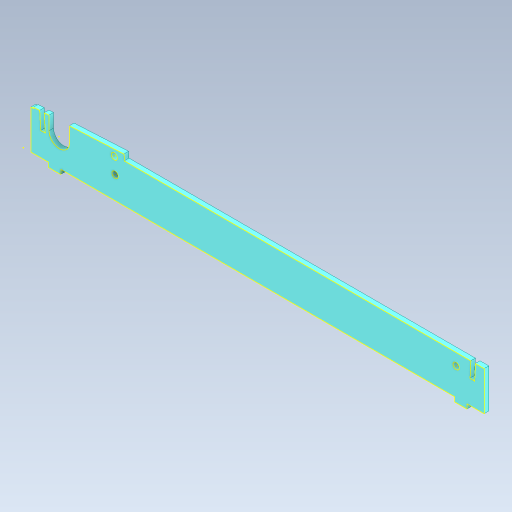
# Autodesk Inventor part: 零件1
Saved by Autodesk Inventor 2023 (Build 270158000, 158)
## iProperties
Created: 2023-04-16
Part Number: 零件1
Material: 一般
Document SubType Name: Modeling
Designer: JOU
Density: 1 g/cm^3
Appearance: 預設
Author: JOU
Autodesk Inventor part; units mm, degrees
ref_plane "YZ Plane" through (0, 0, 0) normal (1, 0, 0) x (0, 1, 0)
ref_plane "XZ Plane" through (0, 0, 0) normal (0, 1, 0) x (-1, 0, 0)
ref_plane "XY Plane" through (0, 0, 0) normal (0, 0, 1) x (1, 0, 0)
sketch "草圖1" plane through (0, 0, 0) normal (0, 0, 1) x (1, 0, 0)
  line L0 (0, 25) -> (300, 25)
  line L1 (300, 25) -> (300, 0)
  line L2 (300, 0) -> (0, 0)
  line L3 (0, 0) -> (0, 25)
  circle A0 centre (23, 17.5) radius 6.55
  circle A1 centre (277, 17.5) radius 2
  line L4 (16, 0) -> (24, 0)
  line L5 (24, 0) -> (24, -2.9)
  line L6 (24, -2.9) -> (16, -2.9)
  line L7 (16, -2.9) -> (16, 0)
  line L8 (276, 0) -> (284, 0)
  line L9 (284, 0) -> (284, -2.9)
  line L10 (284, -2.9) -> (276, -2.9)
  line L11 (276, -2.9) -> (276, 0)
  line L12 (0, 25) -> (5, 25)
  line L13 (5, 25) -> (5, 0)
  line L14 (5, 0) -> (0, 0)
  line L15 (0, 0) -> (0, 25)
  line L16 (300, 25) -> (295, 25)
  line L17 (295, 25) -> (295, 0)
  line L18 (295, 0) -> (300, 0)
  line L19 (300, 0) -> (300, 25)
  line L20 (24, -1.45) -> (276, -1.45) construction
  point P0 (16, -1.45)
  point P1 (284, -1.45)
  point P2 (284, 0)
  point P3 (24, 0)
  point P4 (150, -1.45)
  point P5 (150, 0)
  dimension "d0" = 300
  dimension "d1" = 25
  dimension "d2" = 7.5
  dimension "d3" = 13.1
  dimension "d4" = 23
  dimension "d5" = 23
  dimension "d6" = 7.5
  dimension "d7" = 4
  dimension "d12" = 8
  dimension "d13" = 2.9
  dimension "d14" = 8
  dimension "d30" = 5
  dimension "d31" = 5
  dimension "d32" = 252
  constraints: 42 end point, 10 parallel, 6 midpoint, 5 horizontal, 5 perpendicular, 5 point on line, 2 centre point, 1 coincident, 1 vertical alignment
  measures "d0" distance of L0.start L0.end
  measures "d1" distance of L2.end L0.start
  measures "d2" distance from line of L0 A0.centre
  measures "d3" diameter of A0
  measures "d4" distance from line of L3 A0.centre
  measures "d5" distance from line of A1.centre L1
  measures "d6" distance from line of L0 A1.centre
  measures "d7" diameter of A1
  measures "d12" distance of L5.end L6.end
  measures "d13" distance of L4.end L5.end
  measures "d14" distance of L9.end L10.end
  measures "d30" distance between parallel lines of L3 L13
  measures "d31" distance between parallel lines of L1 L17
  measures "d32" distance from line of L20.start L11
extrude "擠出1" add sketch "草圖1" along normal blind 3 contours L0 L17 L2 L13 | L2 L5 L6 L7 | L9 L10 L11 L2
sketch "草圖2" plane through (0, 0, 3) normal (0, 0, 1) x (1, 0, 0)
  line L0 (10.5404, 25) -> (13.4864, 25.1544)
  line L1 (13.4864, 25.1544) -> (14.0097, 15.1681)
  line L2 (14.0097, 15.1681) -> (11.0638, 15.0137)
  line L3 (11.0638, 15.0137) -> (10.5404, 25)
  line L4 (295, 25) -> (5, 25) projected
  line L5 (16.048, 25) -> (29.13, 25.6856)
  line L6 (29.13, 25.6856) -> (30.1465, 6.2887)
  line L7 (30.1465, 6.2887) -> (17.0645, 5.6031)
  line L8 (17.0645, 5.6031) -> (16.048, 25)
  circle A0 centre (23, 17.5) radius 6.55 projected
  line L9 (14.0097, 15.1681) -> (16.5562, 15.3016)
  line L10 (286.4135, 25.1544) -> (289.3595, 25)
  line L11 (289.3595, 25) -> (288.8361, 15.0137)
  line L12 (288.8361, 15.0137) -> (285.8901, 15.1681)
  line L13 (285.8901, 15.1681) -> (286.4135, 25.1544)
  line L14 (275.2453, 22.2337) -> (279.2399, 22.0243)
  line L15 (279.2399, 22.0243) -> (278.6818, 11.3762)
  line L16 (278.6818, 11.3762) -> (274.6873, 11.5855)
  line L17 (274.6873, 11.5855) -> (275.2453, 22.2337)
  circle A1 centre (277, 17.5) radius 2 projected
  line L18 (285.8901, 15.1681) -> (278.8997, 15.5344)
  point P0 (0, 0)
  point P1 (300, 25)
  point P2 (0, 25)
  point P3 (286.4054, 25)
  point P4 (13.4945, 25)
  dimension "d16" = 2.95
  dimension "d18" = 10
  dimension "d19" = 87
  dimension "d20" = 87
  dimension "d22" = 87
  dimension "d23" = 87
  dimension "d24" = 2.95
  dimension "d25" = 10
  dimension "d33" = 9.1
  dimension "d34" = 9
  constraints: 36 end point, 8 parallel, 6 perpendicular, 4 point on line, 4 tangent, 1 midpoint
  measures "d16" distance of L0.start L0.end
  measures "d18" distance of L0.end L1.end
  measures "d19" angle of L1 L4
  measures "d20" angle of L6 L4
  measures "d22" angle of L4 L17
  measures "d23" angle of L4 L13
  measures "d24" distance of L10.start L10.end
  measures "d25" distance of L10.end L11.end
  measures "d33" distance from line of L1 A0.centre
  measures "d34" distance from line of L13 A1.centre
extrude "擠出2" cut sketch "草圖2" against normal up to surface (3 mm away) contours L4 L1 L2 L3 | L11 L12 L13 L4
sketch "草圖7" plane through (0, 0, 3) normal (0, 0, 1) x (1, 0, 0)
  line L0 (64.4714, 28.6858) -> (65.4135, 10.7104)
  line L1 (65.4135, 10.7104) -> (7.493, 7.675)
  line L2 (7.493, 7.675) -> (6.5509, 25.6503)
  line L3 (6.5509, 25.6503) -> (64.4714, 28.6858)
  line L4 (13.4945, 25) -> (14.0097, 15.1681) projected
  circle A0 centre (23, 17.5) radius 6.55 projected
  line L5 (285.8901, 15.1681) -> (286.4054, 25) projected
  line L6 (286.4054, 25) -> (13.4945, 25) projected
  line L7 (13.4945, 25) -> (14.0097, 15.1681) projected
  line L8 (14.0097, 15.1681) -> (11.0638, 15.0137) projected
  line L9 (11.0638, 15.0137) -> (10.5404, 25) projected
  line L10 (10.5404, 25) -> (5, 25) projected
  line L11 (5, 25) -> (5, 0) projected
  line L12 (5, 0) -> (16, 0) projected
  line L13 (16, 0) -> (16, -2.9) projected
  line L14 (16, -2.9) -> (24, -2.9) projected
  line L15 (24, -2.9) -> (24, 0) projected
  line L16 (24, 0) -> (276, 0) projected
  line L17 (276, 0) -> (276, -2.9) projected
  line L18 (276, -2.9) -> (284, -2.9) projected
  line L19 (284, -2.9) -> (284, 0) projected
  line L20 (284, 0) -> (295, 0) projected
  line L21 (295, 0) -> (295, 25) projected
  line L22 (295, 25) -> (289.3595, 25) projected
  line L23 (289.3595, 25) -> (288.8361, 15.0137) projected
  line L24 (288.8361, 15.0137) -> (285.8901, 15.1681) projected
  circle A1 centre (23, 17.5) radius 6.55 projected
  circle A2 centre (277, 17.5) radius 2 projected
  line L25 (13.4945, 25) -> (13.4414, 26.0114)
  line L26 (10.5404, 25) -> (11.0638, 15.0137) projected
  line L27 (10.5404, 25) -> (10.4955, 25.857)
  point P0 (0, 0)
  point P1 (64.6646, 25)
  point P2 (6.585, 25)
  dimension "d50" = 42
  dimension "d51" = 16
  dimension "d52" = 18
  dimension "d53" = 9
  constraints: 12 end point, 4 parallel, 2 point on line, 1 collinear, 1 perpendicular
  measures "d50" distance from line of L0 A0.centre
  measures "d51" distance from line of L2 A0.centre
  measures "d52" distance of L0.start L0.end
  measures "d53" distance from line of A0.centre L1
extrude "擠出5" add sketch "草圖7" against normal up to surface (3 mm away) contours L0 L6 L25 L3 | L27 L10 L2 L3
sketch "草圖9" plane through (0, 0, 3) normal (0, 0, 1) x (1, 0, 0)
  line L0 (10.4955, 25.857) -> (6.5509, 25.6503) projected
  line L1 (6.5509, 25.6503) -> (64.4714, 28.6858)
  line L2 (64.4714, 28.6858) -> (65.4135, 10.7104)
  line L3 (65.4135, 10.7104) -> (7.493, 7.675)
  line L4 (7.493, 7.675) -> (6.5509, 25.6503)
  circle A0 centre (58.1897, 24.3511) radius 2
  circle A1 centre (58.713, 14.3648) radius 2
  line L5 (58.1897, 24.3511) -> (58.713, 14.3648)
  line L6 (58.4513, 19.3579) -> (64.9424, 19.6981)
  circle A2 centre (23, 17.5) radius 6.55 projected
  point P0 (0, 0)
  dimension "d60" = 18
  dimension "d64" = 4
  dimension "d66" = 6.5
  dimension "d67" = 10
  constraints: 12 end point, 3 perpendicular, 2 centre point, 2 midpoint, 2 parallel, 1 collinear, 1 equal radius
  measures "d60" distance of L1.end L2.end
  measures "d64" diameter of A0
  measures "d66" distance of L6.start L6.end
  measures "d67" distance of L5.start L5.end
extrude "擠出6" cut sketch "草圖9" against normal up to surface (3 mm away) contours A0 | A1
sketch "草圖11" plane through (0, 0, 3) normal (0, 0, 1) x (1, 0, 0)
  line L0 (16.45, 26.8556) -> (29.55, 26.8556)
  line L1 (29.55, 26.8556) -> (29.55, 17.5)
  line L2 (29.55, 17.5) -> (16.45, 17.5)
  line L3 (16.45, 17.5) -> (16.45, 26.8556)
  circle A0 centre (23, 17.5) radius 6.55 projected
  line L4 (64.4714, 28.6858) -> (13.4414, 26.0114) projected
  point P0 (0, 0)
  dimension "d74" = 13.1
  constraints: 8 end point, 2 parallel, 2 point on circle, 1 horizontal, 1 perpendicular, 1 point on line
  measures "d74" distance of L1.end L2.end
extrude "擠出7" cut sketch "草圖11" against normal blind 10 contours L0 L4 L3 | L1 A0 L3 L4 | L2 A0 picked at (21.0033, 19.0372)
sketch "草圖10" plane through (0, 0, 3) normal (0, 0, 1) x (1, 0, 0)
  circle A0 centre (58.1897, 24.3511) radius 2 projected
  circle A1 centre (58.713, 14.3648) radius 2 projected
  line L0 (285.8901, 15.1681) -> (286.4054, 25) projected
  line L1 (286.4054, 25) -> (64.6646, 25) projected
  line L2 (64.6646, 25) -> (64.4714, 28.6858) projected
  line L3 (64.4714, 28.6858) -> (29.55, 26.8556) projected
  line L4 (13.4414, 26.0114) -> (14.0097, 15.1681) projected
  line L5 (14.0097, 15.1681) -> (11.0638, 15.0137) projected
  line L6 (11.0638, 15.0137) -> (10.4955, 25.857) projected
  line L7 (10.4955, 25.857) -> (6.5509, 25.6503) projected
  line L8 (6.5509, 25.6503) -> (6.585, 25) projected
  line L9 (6.585, 25) -> (5, 25) projected
  line L10 (5, 25) -> (5, 0) projected
  line L11 (5, 0) -> (16, 0) projected
  line L12 (16, 0) -> (16, -2.9) projected
  line L13 (16, -2.9) -> (24, -2.9) projected
  line L14 (24, -2.9) -> (24, 0) projected
  line L15 (24, 0) -> (276, 0) projected
  line L16 (276, 0) -> (276, -2.9) projected
  line L17 (276, -2.9) -> (284, -2.9) projected
  line L18 (284, -2.9) -> (284, 0) projected
  line L19 (284, 0) -> (295, 0) projected
  line L20 (295, 0) -> (295, 25) projected
  line L21 (295, 25) -> (289.3595, 25) projected
  line L22 (289.3595, 25) -> (288.8361, 15.0137) projected
  line L23 (288.8361, 15.0137) -> (285.8901, 15.1681) projected
  arc A2 (16.45, 17.5) -> (29.55, 17.5) centre (23, 17.5) ccw projected
  circle A3 centre (277, 17.5) radius 2 projected
  line L24 (29.55, 26.8556) -> (29.55, 17.5) projected
  line L25 (16.45, 17.5) -> (16.45, 26.1691) projected
  line L26 (16.45, 26.1691) -> (13.4414, 26.0114) projected
  point P0 (0, 0)
equation "\"d20\" = d19"
equation "\"d22\" = d23"
